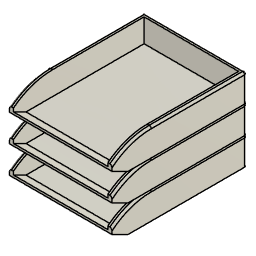
Paperstorage-V2 (Autodesk Fusion 360 design; units mm, degrees)
Autodesk Fusion 360 part; units mm, degrees
sketch "Skizze1" plane through (0, 0, 0) normal (0, 0, 1) x (1, 0, 0)
  line L0 (-15, 30) -> (240, 30)
  line L1 (240, 30) -> (240, -305)
  line L2 (240, -305) -> (-15, -305)
  line L3 (-15, -305) -> (-15, 30)
  dimension "d1" = 255
  dimension "d2" = 335
  constraint horizontal L0
  constraint vertical L1
  constraint horizontal L2
  constraint vertical L3
  measures "d1" distance of L0.start L0.end
  measures "d2" distance of L0.start L2.end
sketch "Skizze2" plane through (0, -305, 0) normal (0, -1, 0) x (1, 0, 0)
  line L0 (-15, 0) -> (240, 0)
  line L1 (240, 0) -> (240, 205)
  line L2 (240, 205) -> (-15, 205)
  line L3 (-15, 205) -> (-15, 0)
sketch "Skizze3" plane through (0, -305, 0) normal (0, -1, 0) x (1, 0, 0)
  line L0 (-5, 205) -> (-15, 205)
  line L1 (-15, 205) -> (-15, 0)
  line L2 (-15, 0) -> (-5, 0)
  line L3 (-5, 0) -> (-5, 205)
  line L4 (230, 0) -> (240, 0)
  line L5 (240, 0) -> (240, 205)
  line L6 (240, 205) -> (230, 205)
  line L7 (230, 205) -> (230, 0)
  line L8 (-5, 0) -> (230, 0)
  line L9 (230, 0) -> (230, 18)
  line L10 (230, 18) -> (-5, 18)
  line L11 (-5, 18) -> (-5, 0)
  line L12 (-5, 68) -> (230, 68)
  line L13 (230, 68) -> (230, 86)
  line L14 (230, 86) -> (-5, 86)
  line L15 (-5, 86) -> (-5, 68)
  line L16 (-5, 154) -> (230, 154)
  line L17 (230, 154) -> (230, 136)
  line L18 (230, 136) -> (-5, 136)
  line L19 (-5, 136) -> (-5, 154)
  line L20 (240, 205) -> (-15, 205)
  dimension "d8" = 235
  dimension "d9" = 10
  dimension "d12" = 10
  dimension "d13" = 205
  dimension "d14" = 18
  dimension "d15" = 50
  dimension "d16" = 18
  dimension "d17" = 50
  dimension "d18" = 18
  dimension "d19" = 51
  constraint horizontal L0
  constraint vertical L1
  constraint horizontal L2
  constraint vertical L3
  constraint horizontal L4
  constraint vertical L5
  constraint horizontal L6
  constraint vertical L7
  constraint horizontal L8
  constraint vertical L9
  constraint horizontal L10
  constraint vertical L11
  constraint coincident L7 L9.end
  constraint horizontal L12
  constraint vertical L13
  constraint horizontal L14
  constraint vertical L15
  constraint coincident L7 L13.end
  constraint horizontal L16
  constraint vertical L17
  constraint horizontal L18
  constraint vertical L19
  constraint coincident L7 L17.end
  constraint coincident L3 L16.start
  measures "d8" distance of L3 L7
  measures "d9" distance of L4.start L4.end
  measures "d12" distance of L1.end L2.end
  measures "d13" distance of L4.start L6.end
  measures "d14" distance of L2.end L10.end
  measures "d15" distance of L10 L12
  measures "d16" distance of L12.start L14.end
  measures "d17" distance of L14 L18
  measures "d18" distance of L16 L18
  measures "d19" distance of L16 L20
sketch "Skizze4" plane through (0, 0, 0) normal (0, 0, 1) x (1, 0, 0)
  line L0 (370, 20) -> (625, 20)
  line L1 (625, 20) -> (625, -315)
  line L2 (625, -315) -> (370, -315)
  line L3 (370, -315) -> (370, 20)
  dimension "d22" = 255
  dimension "d23" = 335
  constraint horizontal L0
  constraint vertical L1
  constraint horizontal L2
  constraint vertical L3
  measures "d22" distance of L0.start L0.end
  measures "d23" distance of L0.start L2.end
extrude "Extrusion3" add sketch "Skizze4" along normal blind 68 makes body 1
sketch "Skizze5" plane through (625, 0, 0) normal (1, 0, 0) x (0, 1, 0)
  line L0 (-315, 0) -> (20, 0)
  line L1 (20, 0) -> (20, 68)
  line L2 (20, 68) -> (-315, 68)
  line L3 (-315, 68) -> (-315, 0)
  line L4 (-275, 0) -> (-315, 20)
  line L5 (-315, 20) -> (-315, 34)
  arc A0 (-217.2794, 68) -> (-315, 34) centre (-217.2794, -89.4311) ccw
  constraint coincident L0 L4.start
  constraint coincident L3 L4.end
  constraint midpoint L3 L5.end
  constraint tangent L2 A0
  constraint coincident L2 A0.start
extrude "Extrusion4" cut sketch "Skizze5" against normal blind 270 contours L0 L3 L4 | L2 L3 A0 bodies 1
sketch "Skizze6" plane through (0, 0, 68) normal (0, 0, 1) x (-1, 0, 0)
  line L0 (-370, 217.2794) -> (-625, 217.2794)
  line L1 (-625, 217.2794) -> (-625, -20)
  line L2 (-625, -20) -> (-370, -20)
  line L3 (-370, -20) -> (-370, 217.2794)
  line L4 (-380, -10) -> (-615, -10)
  line L5 (-615, -10) -> (-615, 329.167)
  line L6 (-615, 329.167) -> (-380, 329.167)
  line L7 (-380, 329.167) -> (-380, -10)
  line L8 (-625, 315) -> (-625, 217.2794)
  line L9 (-370, 315) -> (-370, -20)
  line L10 (-370, -20) -> (-625, -20)
  dimension "d28" = 10
  dimension "d29" = 10
  dimension "d30" = 10
  constraint horizontal L4
  constraint vertical L5
  constraint horizontal L6
  constraint vertical L7
  measures "d28" distance of L5 L8
  measures "d29" distance of L7 L9
  measures "d30" distance of L4 L10
extrude "Extrusion5" cut sketch "Skizze6" against normal blind 58 contours L0 L4 L5 L7 | L0 L5 L6 L7 bodies 1
sketch "Skizze7" plane through (380, 0, 0) normal (1, 0, 0) x (0, 1, 0)
  line L0 (-315, 20) -> (-295, 10)
  line L1 (-295, 10) -> (10, 10)
  line L2 (10, 10) -> (10, 68)
  line L3 (10, 68) -> (-217.2794, 68)
  arc A0 (-217.2794, 68) -> (-315, 34) centre (-217.2794, -89.4311) ccw
  line L4 (-315, 34) -> (-315, 20)
  line L5 (-315, 20) -> (-315, 25.5902)
  line L6 (-315, 25.5902) -> (-283.8197, 10)
  line L7 (-275, 0) -> (-315, 20)
  dimension "d33" = 5
  dimension "d34" = 5
  constraint coincident L0.start L4.end
  constraint coincident L4 L5.end
  constraint perpendicular L1 L5
  constraint coincident L1 L6.end
  measures "d33" distance of L6 L7
  measures "d34" distance of L6 L7
extrude "Extrusion6" add sketch "Skizze7" along normal blind 235 contours L0 L1 L4 L5 L6 L7 bodies 1
fillet "Abrundung1" radius 5 2 edges at (625, -269.0126, 59.2572) (625, -98.6397, 68) on bodies 1
fillet "Abrundung2" radius 5 5 edges at (625, 20, 31.5) (623.5355, 20, 66.5355) (495, 20, 68) (370, -98.6397, 68) (370, -269.0126, 59.2572) on bodies 1
copy_body "Körper kopieren/einfügen1" bodies 1 makes body 2
move_body "Verschieben1" bodies 2 to x (1, 0, 0) y (0, 1, 0) z (0, 0, 1) at (0, 0, 68)
copy_body "Körper kopieren/einfügen2" bodies 1 makes body 3
move_body "Verschieben2" bodies 3 to x (1, 0, 0) y (0, 1, 0) z (0, 0, 1) at (0, 0, 136)
named bodies: "storage-1", "storage-2", "storage-3"
